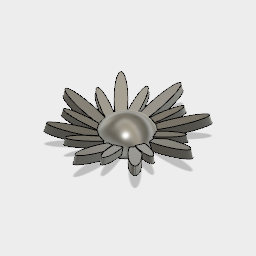
flower (Autodesk Fusion 360 design; units mm, degrees)
Autodesk Fusion 360 part; units mm, degrees
sketch "草图1" plane through (0, 0, 0) normal (0, 1, 0) x (1, 0, 0)
  ellipse E0 centre (-30, -25) end of major axis (-20, -25) minor radius 2
  line L0 (-40, -25) -> (-20, -25)
  line L1 (-30, -27) -> (-30, -23)
  dimension "d1" = 4
extrude "拉伸1" add sketch "草图1" along normal blind 3 makes body 1
move_body "移动1" bodies 1 to x (0.965926, 0.258819, 0) y (-0.258819, 0.965926, 0) z (0, 0, 1) at (-1.0222, 7.7646, 0)
move_body "移动5" bodies 1 to x (1, 0, 0) y (0, 1, 0) z (0, 0, 1) at (0.1029, 2.6075, 0)
pattern_circular "C-阵列1" count 8 over 360 about axis through (-44.5389, 3.9875, 27.0101) along (0, -1, 0) of bodies 1 makes body 2 at (-33.8206, 3.7663, 32.1863) makes body 3 at (-40.6197, 3.7679, 38.2553) makes body 4 at (-50.9148, 3.2046, 39.0282) makes body 5 at (-55.7841, 3.7679, 30.9292) makes body 6 at (-55.2571, 3.7663, 21.8338) makes body 7 at (-48.5287, 4.1721, 14.2565) makes body 8 at (-38.1629, 3.2046, 14.9919)
copy_body "复制和粘贴实体1" bodies 1 2 3 4 5 6 7 8 makes body 9 makes body 10 makes body 11 makes body 12 makes body 13 makes body 14 makes body 15 makes body 16
scale "缩放1" factor 0.8 about (-46.0917, 2.9171, 31.4055) bodies 12 13 11 10 14 15 16 9
move_body "移动7" bodies 9 10 11 12 13 14 15 16 to x (0.906308, 0, 0.422618) y (0, 1, 0) z (-0.422618, 0, 0.906308) at (7.242, 0, 21.3536)
sphere "球体基本要素1" add diameter 20 placed x (1, 0, 0) y (0, 0, -1) z (0, 1, 0) at (-5, 0, 25) separate body makes body 17
move_body "移动8" bodies 17 to x (1, 0, 0) y (0, 1, 0) z (0, 0, 1) at (-39.8903, -1.0138, 1.9956)
combine "合并1" operation add target body 17 tool bodies 7
combine "合并2" operation add target body 17 tool bodies 15 8 16 1 9 2 10 3 11 4 12 5 13 6 14
box "长方体基本要素2" add length 50 width 50 height -20 placed x (0, 0, -1) y (-1, 0, 0) z (0, 1, 0) at (40, 0, 72) separate body makes body 18
move_body "移动9" bodies 18 to x (1, 0, 0) y (0, 1, 0) z (0, 0, 1) at (-59.5062, 0.7096, -19.9221)
combine "合并3" operation cut target body 17 tool bodies 18
